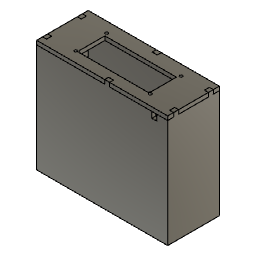
NXP_CUP_TIMER v4 (Autodesk Fusion 360 design; units mm, degrees)
Autodesk Fusion 360 part; units mm, degrees
note: some values were not read from the file. Set by a fixed rule: which sketch regions a step uses.
sketch "Sketch1" plane through (0, 0, 0) normal (0, 0, 1) x (1, 0, 0)
  line L0 (-40, 18) -> (40, 18)
  circle A0 centre (37.5, -15.5) radius 2.4
  line L1 (36, -15.3) -> (36, 12.2)
  circle A1 centre (-37.5, 15.5) radius 1.4
  circle A2 centre (-37.5, -15.5) radius 1.4
  line L2 (36, 12.2) -> (-36, 12.2)
  circle A3 centre (-37.5, -15.5) radius 2.4
  line L3 (-33.5216, 18) -> (8, 18)
  line L4 (40, 18) -> (40, -18)
  line L5 (-36, 12.2) -> (-36, -15.3)
  circle A4 centre (37.5, 15.5) radius 1.4
  circle A5 centre (-37.5, 15.5) radius 2.4
  circle A6 centre (37.5, -15.5) radius 1.4
  line L6 (-33.5216, 14) -> (-33.5216, 18)
  line L7 (40, -18) -> (-40, -18)
  line L8 (8, 18) -> (8, 14)
  line L9 (8, 14) -> (-33.5216, 14)
  line L10 (-36, -15.3) -> (36, -15.3)
  circle A7 centre (37.5, 15.5) radius 2.4
  line L11 (-40, -18) -> (-40, 18)
  dimension "d1" = 2.8
  dimension "d2" = 4.8
  dimension "d3" = 2.8
  dimension "d4" = 4.8
  dimension "d5" = 2.8
  dimension "d6" = 4.8
  dimension "d7" = 2.8
  dimension "d8" = 4.8
  constraint concentric A1 A5
  constraint concentric A2 A3
  constraint concentric A4 A7
  constraint concentric A0 A6
  constraint horizontal L0
  constraint vertical L4
  constraint horizontal L7
  constraint vertical L11
  constraint horizontal L3
  constraint vertical L8
  constraint horizontal L9
  constraint vertical L6
  constraint coincident L3.start L0
  constraint horizontal L10
  constraint vertical L1
  constraint horizontal L2
  constraint vertical L5
  measures "d1" diameter of A1
  measures "d2" diameter of A5
  measures "d3" diameter of A2
  measures "d4" diameter of A3
  measures "d5" diameter of A4
  measures "d6" diameter of A7
  measures "d7" diameter of A6
  measures "d8" diameter of A0
sketch "Sketch2" plane through (0, 0, 0) normal (0, 0, 1) x (1, 0, 0)
  line L0 (55, 20) -> (-5, 20)
  line L1 (-5, 20) -> (-5, -20)
  line L2 (-5, -20) -> (55, -20)
  line L3 (55, -20) -> (55, 20)
  line L4 (61, 26) -> (-71, 26)
  line L5 (-71, 26) -> (-71, -26)
  line L6 (-71, -26) -> (61, -26)
  line L7 (61, -26) -> (61, 26)
  line L8 (57, 22) -> (-67, 22)
  line L9 (-67, 22) -> (-67, -22)
  line L10 (-67, -22) -> (57, -22)
  line L11 (57, -22) -> (57, 22)
  line L12 (-39.9718, 26) -> (-45, 26)
  line L13 (-45, 26) -> (-45, -26)
  line L14 (-45, -26) -> (-39.9718, -26)
  line L15 (-39.9718, -26) -> (-39.9718, 26)
  line L16 (-20, 13) -> (-30, 13)
  line L17 (-30, 13) -> (-30, -13)
  line L18 (-30, -13) -> (-20, -13)
  line L19 (-20, -13) -> (-20, 13)
  dimension "d15" = 60
  dimension "d16" = 40
  dimension "d19" = 132
  dimension "d20" = 52
  dimension "d22" = 26
  constraint horizontal L0
  constraint vertical L1
  constraint horizontal L2
  constraint vertical L3
  constraint horizontal L4
  constraint vertical L5
  constraint horizontal L6
  constraint vertical L7
  constraint horizontal L8
  constraint vertical L9
  constraint horizontal L10
  constraint vertical L11
  constraint horizontal L12
  constraint vertical L13
  constraint horizontal L14
  constraint vertical L15
  constraint coincident L6 L13.end
  constraint coincident L4 L12.start
  constraint horizontal L16
  constraint vertical L17
  constraint horizontal L18
  constraint vertical L19
  measures "d15" distance of L0.start L0.end
  measures "d16" distance of L0.start L2.end
  measures "d19" distance of L4.start L4.end
  measures "d20" distance of L4.start L6.end
  measures "d22" distance of L16.start L18.end
extrude "Extrude1" add sketch "Sketch2" along normal blind 4 contours L0 L1 L2 L3 | L4 L6 L7 L8 L10 L11 L15 | L4 L8 L12 L13 L15 | L4 L5 L6 L8 L9 L10 L13 | L8 L10 L13 L15 | L8 L10 L11 L15 | L6 L10 L13 L14 L15 | L8 L9 L10 L13 | L16 L17 L18 L19 makes body 1
extrude "Extrude2" add sketch "Sketch2" along normal blind 109 contours L4 L6 L7 L8 L10 L11 L15 | L4 L8 L12 L13 L15 | L4 L5 L6 L8 L9 L10 L13 | L6 L10 L13 L14 L15 bodies 1
extrude "Extrude3" add sketch "Sketch2" along normal blind 74 contours L8 L10 L13 L15 bodies 1
sketch "Sketch3" plane through (-71, 0, 0) normal (-1, 0, 0) x (0, -1, 0)
  line L0 (-26, 0) -> (26, 0)
  line L1 (26, 0) -> (26, 109)
  line L2 (26, 109) -> (-26, 109)
  line L3 (-26, 109) -> (-26, 0)
  line L4 (-11, 95) -> (11, 95)
  line L5 (11, 95) -> (11, 28)
  line L6 (11, 28) -> (-11, 28)
  line L7 (-11, 28) -> (-11, 95)
  circle A0 centre (-11, 28) radius 2.1
  circle A1 centre (-11, 95) radius 2.1
  circle A2 centre (11, 95) radius 2.1
  circle A3 centre (11, 28) radius 2.1
  dimension "d31" = 22
  dimension "d32" = 67
  dimension "d33" = 4.2
  dimension "d34" = 4.2
  dimension "d35" = 4.2
  dimension "d36" = 4.2
  constraint horizontal L4
  constraint vertical L5
  constraint horizontal L6
  constraint vertical L7
  constraint coincident L6.end L7.start
  constraint coincident L4.start L7.end
  constraint coincident L4.end L5.start
  constraint coincident L5.end L6.start
  measures "d31" distance of L4.start L4.end
  measures "d32" distance of L4.start L6.end
  measures "d33" diameter of A0
  measures "d34" diameter of A1
  measures "d35" diameter of A2
  measures "d36" diameter of A3
sketch "Sketch4" plane through (0, 0, 109) normal (0, 0, 1) x (-1, 0, 0)
  line L0 (-57, -22) -> (-57, 22)
  line L1 (-57, 22) -> (67, 22)
  line L2 (67, 22) -> (67, -22)
  line L3 (67, -22) -> (-57, -22)
  line L4 (71, 26) -> (-61, 26)
  line L5 (-61, 26) -> (-61, -26)
  line L6 (-61, -26) -> (71, -26)
  line L7 (71, -26) -> (71, 26)
  line L8 (-61, 26) -> (71, 26)
  line L9 (71, 26) -> (71, -26)
  line L10 (71, -26) -> (-61, -26)
  line L11 (-61, -26) -> (-61, 26)
  line L12 (67, 20) -> (71, 20)
  line L13 (71, 20) -> (71, 15)
  line L14 (71, 15) -> (67, 15)
  line L15 (67, 15) -> (67, 20)
  line L16 (71, -20) -> (67, -20)
  line L17 (67, -20) -> (67, -15)
  line L18 (67, -15) -> (71, -15)
  line L19 (71, -15) -> (71, -20)
  line L20 (-57, 20) -> (-61, 20)
  line L21 (-61, 20) -> (-61, 15)
  line L22 (-61, 15) -> (-57, 15)
  line L23 (-57, 15) -> (-57, 20)
  line L24 (-57, -20) -> (-61, -20)
  line L25 (-61, -20) -> (-61, -15)
  line L26 (-61, -15) -> (-57, -15)
  line L27 (-57, -15) -> (-57, -20)
  line L28 (2.5, -22) -> (-2.5, -22)
  line L29 (-2.5, -22) -> (-2.5, -26)
  line L30 (-2.5, -26) -> (2.5, -26)
  line L31 (2.5, -26) -> (2.5, -22)
  line L32 (2.5, 22) -> (-2.5, 22)
  line L33 (-2.5, 22) -> (-2.5, 26)
  line L34 (-2.5, 26) -> (2.5, 26)
  line L35 (2.5, 26) -> (2.5, 22)
  circle A0 centre (-33.0216, 15.5) radius 2.4
  line L36 (-35.5216, -18) -> (-35.5216, 18)
  circle A1 centre (-33.0216, -15.5) radius 2.4
  line L37 (38, -14) -> (38, -18)
  line L38 (-31.5216, -12.2) -> (40.4784, -12.2)
  line L39 (44.4784, -18) -> (-35.5216, -18)
  line L40 (38, -18) -> (-3.5216, -18)
  line L41 (-3.5216, -18) -> (-3.5216, -14)
  circle A2 centre (-33.0216, 15.5) radius 1.4
  line L42 (-31.5216, 15.3) -> (-31.5216, -12.2)
  circle A3 centre (-33.0216, -15.5) radius 1.4
  line L43 (44.4784, 18) -> (44.4784, -18)
  circle A4 centre (41.9784, 15.5) radius 2.4
  line L44 (40.4784, 15.3) -> (-31.5216, 15.3)
  circle A5 centre (41.9784, 15.5) radius 1.4
  circle A6 centre (41.9784, -15.5) radius 2.4
  line L45 (40.4784, -12.2) -> (40.4784, 15.3)
  line L46 (-35.5216, 18) -> (44.4784, 18)
  circle A7 centre (41.9784, -15.5) radius 1.4
  line L47 (-3.5216, -14) -> (38, -14)
  line L48 (-50, 26) -> (-45, 26)
  line L49 (-45, 26) -> (-45, 22)
  line L50 (-45, 22) -> (-50, 22)
  line L51 (-50, 22) -> (-50, 26)
  point P0 (4.4784, 0)
  point P1 (4.4784, 0)
  dimension "d37" = 5
  dimension "d38" = 4
  dimension "d39" = 5
  dimension "d44" = 2.8
  dimension "d45" = 4.8
  dimension "d46" = 2.8
  dimension "d47" = 4.8
  dimension "d48" = 2.8
  dimension "d49" = 4.8
  dimension "d50" = 2.8
  dimension "d51" = 4.8
  constraint horizontal L8
  constraint vertical L9
  constraint horizontal L10
  constraint vertical L11
  constraint coincident L6.end L7.start
  constraint coincident L4.end L5.start
  constraint horizontal L12
  constraint vertical L13
  constraint horizontal L14
  constraint vertical L15
  constraint coincident L7 L13.end
  constraint coincident L2 L12.start
  constraint horizontal L16
  constraint vertical L17
  constraint horizontal L18
  constraint vertical L19
  constraint coincident L2 L17.end
  constraint coincident L7 L16.start
  constraint horizontal L20
  constraint vertical L21
  constraint horizontal L22
  constraint vertical L23
  constraint coincident L11 L21.end
  constraint coincident L0 L20.start
  constraint horizontal L24
  constraint vertical L25
  constraint horizontal L26
  constraint vertical L27
  constraint coincident L5 L25.end
  constraint coincident L0 L24.start
  constraint horizontal L28
  constraint vertical L29
  constraint horizontal L30
  constraint vertical L31
  constraint coincident L3 L28.start
  constraint horizontal L32
  constraint vertical L33
  constraint horizontal L34
  constraint vertical L35
  constraint coincident L1 L32.start
  constraint concentric A6 A7
  constraint concentric A4 A5
  constraint concentric A1 A3
  constraint concentric A0 A2
  constraint coincident L37.end L39
  constraint horizontal L48
  constraint vertical L49
  constraint horizontal L50
  constraint vertical L51
  constraint coincident L1 L49.end
  constraint coincident L8 L48.start
  measures "d37" distance of L28.start L28.end
  measures "d38" distance of L28.start L30.end
  measures "d39" distance of L32.start L32.end
  measures "d44" diameter of A7
  measures "d45" diameter of A6
  measures "d46" diameter of A5
  measures "d47" diameter of A4
  measures "d48" diameter of A3
  measures "d49" diameter of A1
  measures "d50" diameter of A2
  measures "d51" diameter of A0
extrude "Extrude4" add sketch "Sketch4" along normal blind 4 contours L0 L5 L11 L24 L25 L26 L27 | L3 L6 L10 L28 L29 L30 L31 | L0 L5 L11 L20 L21 L22 L23 | L2 L7 L9 L16 L17 L18 L19 | L2 L7 L9 L12 L13 L14 L15 | L1 L4 L8 L32 L33 L34 L35 bodies 1
extrude "Extrude5" cut sketch "Sketch2" along normal blind 4 contours L16 L17 L18 L19 bodies 1
extrude "Extrude6" cut sketch "Sketch4" against normal blind 6 contours L1 L4 L8 L48 L49 L50 L51 bodies 1
extrude "Extrude7" add sketch "Sketch4" along normal blind 4 separate body contours L0 L3 L5 L6 L10 L11 L24 L29 | L0 L1 L2 L3 L15 L17 L23 L27 L28 L32 L50 | L0 L5 L11 L22 L26 | L2 L3 L6 L7 L9 L10 L16 L31 | L0 L1 L4 L5 L8 L11 L20 L51 | L2 L7 L9 L14 L18 | L1 L4 L8 L48 L49 L50 L51 | L1 L4 L8 L33 L49 | L1 L2 L4 L7 L8 L9 L12 L35 | A0 L42 L44 | A0 L42 L44 | A4 L44 L45 | A4 L44 L45 | L36 L37 L39 L41 L43 L46 L47 | L37 L39 L40 L41 L47 | A1 | A6 makes body 2
extrude "Extrude8" cut sketch "Sketch3" against normal blind 4 contours L4 L7 A1 | L4 L7 A1 | L4 L5 A2 | L4 L5 A2 | L6 L7 A0 | L6 L7 A0 | L5 L6 A3 | L5 L6 A3 bodies 1
equation "d19 = 126 mm + 6 mm"
equation "d20 = 46 mm + 6 mm"
equation "d25 = 80 mm + 4 mm + 25 mm"
equation "d27 = 70 mm + 4 mm"
named bodies: "CutieTimer", "CapacTimer"
